Autodesk Inventor part; units mm, degrees
(part 2 of 2)
sketch "Sketch52" plane through (68.046336, 24.150723, -1) normal (0, 0.487547, 0.8730967) x (1, 0, 0)
  line L0 (-26.764269, 47.731417) -> (110.67345, 47.731417)
  line L1 (11.777064, 45.962688) -> (24.325703, 45.962688)
  line L2 (24.325703, 9.021095) -> (11.777064, 9.021095)
  line L3 (11.777064, 45.962688) -> (24.325703, 45.962688)
  line L4 (24.325703, 9.021095) -> (11.777064, 9.021095)
  line L5 (14.714671, 39.847676) -> (21.539975, 39.847676)
  line L6 (21.539975, 15.345043) -> (14.712852, 15.345043)
  line L7 (6.346286, 40.416065) -> (11.777064, 45.962688)
  line L8 (24.325703, 45.962688) -> (29.996181, 40.410641)
  line L9 (6.346286, 14.669312) -> (11.777064, 9.021095)
  line L10 (24.325703, 9.021095) -> (29.850784, 14.664032)
  line L11 (12.768778, 17.248514) -> (14.712852, 15.345043)
  line L12 (21.539975, 15.345043) -> (23.571588, 17.250974)
  line L13 (12.768778, 37.860275) -> (14.714671, 39.847676)
  line L14 (21.539975, 39.847676) -> (23.571588, 37.858494)
  line L15 (24.325703, 45.962688) -> (11.777064, 45.962688)
  line L16 (24.675506, 46.319952) -> (30.497659, 40.619399)
  line L17 (5.846286, 40.620088) -> (11.566859, 46.462688)
  line L18 (11.566859, 46.462688) -> (24.529447, 46.462688)
  line L19 (24.529447, 46.462688) -> (24.683636, 46.311992)
  line L20 (15.169294, 5.493045) -> (27.447668, 5.493045)
  line L21 (17.779421, 36.133533) -> (23.071588, 36.133533)
  line L22 (24.529447, 46.462688) -> (33.660701, 37.522418)
  line L23 (5.846286, 14.46793) -> (14.475665, 5.493045)
  line L24 (14.475665, 5.493045) -> (15.169294, 5.493045)
  line L25 (27.447668, 5.493045) -> (33.668767, 11.00658)
  line L26 (40.880024, 36.633533) -> (40.880024, 36.606569)
  line L27 (17.779421, 36.133533) -> (16.268028, 34.718457)
  line L28 (3.760683, 48.300062) -> (70.974232, 48.300062) construction
  line L29 (70.974232, 48.300062) -> (70.974232, 2.785373) construction
  line L30 (70.974232, 2.785373) -> (3.760683, 2.785373) construction
  line L31 (3.760683, 2.785373) -> (3.760683, 48.300062) construction
  line L32 (5.846286, 29.443989) -> (7.926263, 27.407454)
  line L33 (7.926263, 27.407454) -> (5.846286, 25.283108)
  line L34 (27.432742, 27.4203) -> (29.937267, 29.97825)
  line L35 (27.432742, 27.4203) -> (29.909129, 24.995634)
  line L36 (6.346286, 29.654194) -> (8.633331, 27.414916)
  line L37 (5.846286, 40.620088) -> (5.846286, 29.443989)
  line L38 (5.846286, 25.283108) -> (5.846286, 14.46793)
  line L39 (6.346286, 29.654194) -> (6.346286, 40.416065)
  line L40 (6.346286, 14.669312) -> (6.346286, 25.079086)
  line L41 (8.633331, 27.414916) -> (6.346286, 25.079086)
  line L42 (14.714671, 39.847676) -> (21.539975, 39.847676)
  line L43 (21.539975, 15.345043) -> (14.714671, 15.345043)
  line L44 (14.714671, 30.323192) -> (21.539975, 30.323192)
  line L45 (21.539975, 24.068485) -> (14.714671, 24.068485)
  line L46 (14.714671, 30.323192) -> (12.768778, 32.228443)
  line L47 (21.539975, 30.323192) -> (23.571588, 32.398142)
  line L48 (14.714671, 24.068485) -> (12.768778, 22.081084)
  line L49 (21.539975, 24.068485) -> (23.571588, 21.955529)
  line L50 (23.071588, 32.602164) -> (23.071588, 36.133533)
  line L51 (16.268028, 30.823192) -> (21.32977, 30.823192)
  line L52 (21.32977, 30.823192) -> (23.071588, 32.602164)
  line L53 (12.768778, 22.077314) -> (12.768778, 22.081084)
  line L54 (12.768778, 32.228443) -> (12.768778, 32.753075)
  line L55 (12.768778, 17.248514) -> (12.768778, 22.081084)
  line L56 (12.768778, 32.228443) -> (12.768778, 37.860275)
  line L57 (23.571588, 37.858494) -> (23.571588, 32.398142)
  line L58 (23.571588, 21.955529) -> (23.571588, 17.250974)
  line L59 (16.268028, 30.823192) -> (16.268028, 34.718457)
  line L60 (17.779421, 21.258019) -> (23.071588, 21.258019)
  line L61 (17.779421, 21.258019) -> (16.268028, 19.842942)
  line L62 (16.268028, 15.947677) -> (21.32977, 15.947677)
  line L63 (21.32977, 15.947677) -> (23.071588, 17.72665)
  line L64 (16.268028, 15.947677) -> (16.268028, 19.842942)
  line L65 (16.268028, 15.947677) -> (16.268028, 19.842942)
  line L66 (23.071588, 21.258019) -> (23.071588, 17.72665)
  line L67 (31.159581, 23.771299) -> (33.66563, 21.31759)
  line L68 (33.664106, 26.329248) -> (31.159581, 23.771299)
  line L69 (33.668767, 11.00658) -> (33.66563, 21.31759)
  line L70 (33.664106, 26.329248) -> (33.660701, 37.522418)
  line L71 (29.996181, 40.410641) -> (29.937267, 29.97825)
  line L72 (29.909129, 24.995634) -> (29.850784, 14.664032)
  line L73 (43.97433, 21.987313) -> (43.974311, 21.991083)
  line L74 (37.449269, 37.37978) -> (37.449269, 40.416067)
  line L75 (43.909742, 37.37978) -> (37.449269, 37.37978)
  line L76 (36.953115, 37.379779) -> (40.161952, 34.23796)
  line L77 (40.161952, 34.23796) -> (47.408991, 34.23796)
  line L78 (47.408991, 34.753319) -> (47.408991, 34.23796)
  line L79 (47.408991, 34.753319) -> (48.88625, 36.133533)
  line L80 (48.88625, 36.133533) -> (54.178417, 36.133533)
  line L81 (54.178417, 36.133533) -> (54.178417, 32.602164)
  line L82 (54.678417, 37.858494) -> (54.678417, 32.398142)
  line L83 (52.646804, 39.847676) -> (54.678417, 37.858494)
  line L84 (45.8215, 39.847676) -> (52.646804, 39.847676)
  line L85 (43.909742, 37.895138) -> (45.8215, 39.847676)
  line L86 (43.909742, 37.895138) -> (43.909742, 37.37978)
  line L87 (36.953115, 40.620088) -> (36.953115, 37.379779)
  line L88 (36.953115, 40.620088) -> (42.673691, 46.462691)
  line L89 (42.880047, 45.962689) -> (37.449269, 40.416067)
  line L90 (42.673691, 46.462691) -> (55.636273, 46.462691)
  ellipse E0 centre (41.918663, 54.676342) end of major axis (43.418663, 54.676342) minor radius 0.731321
  line L91 (42.880047, 45.962689) -> (55.428686, 45.962689)
  line L92 (26.413444, 60.77068) -> (58.413444, 60.77068)
  line L93 (55.428686, 45.962689) -> (61.099164, 40.410643)
  line L94 (55.636273, 46.462691) -> (64.767394, 37.522279)
  line L95 (61.099164, 40.410643) -> (61.099164, 29.978085)
  line L96 (64.767394, 37.522279) -> (64.767394, 26.329108)
  line L97 (61.099164, 29.978085) -> (55.300317, 23.988246)
  line L98 (64.767394, 26.329108) -> (59.830797, 21.22992)
  line L99 (55.300317, 23.988246) -> (45.910182, 23.988246)
  line L100 (59.830797, 21.22992) -> (48.911426, 21.22992)
  line L101 (45.910182, 23.988246) -> (43.97433, 21.987313)
  line L102 (48.911426, 21.22992) -> (47.471798, 19.741893)
  line L103 (43.97433, 21.987313) -> (43.97433, 17.158512)
  line L104 (47.471798, 19.741893) -> (47.471798, 15.850429)
  line L105 (43.97433, 17.158512) -> (45.918411, 15.25505)
  line L106 (47.471798, 15.850429) -> (61.143322, 15.850429)
  line L107 (61.060189, 15.25505) -> (45.918411, 15.25505)
  line L108 (61.060189, 15.25505) -> (61.060189, 9.021005)
  line L109 (61.143322, 15.850429) -> (64.868674, 12.202883)
  line L110 (64.868674, 12.202883) -> (64.868674, 5.510434)
  line L111 (61.060189, 9.021005) -> (37.453115, 9.021005)
  line L112 (64.868674, 5.510434) -> (40.538917, 5.510434)
  line L113 (69.848141, 4.102168) -> (69.848141, -14.686273)
  line L114 (36.935591, 9.038395) -> (40.538917, 5.510434)
  line L115 (36.935591, 25.300498) -> (36.935591, 9.038395)
  line L116 (37.453115, 25.079086) -> (37.453115, 9.021005)
  line L117 (36.935591, 25.300498) -> (42.433502, 30.823192)
  line L118 (42.673688, 30.323192) -> (37.453115, 25.079086)
  line L119 (42.433502, 30.823192) -> (52.436599, 30.823192)
  line L120 (52.646804, 30.323192) -> (42.673688, 30.323192)
  line L121 (52.436599, 30.823192) -> (54.178417, 32.602164)
  line L122 (54.678417, 32.398142) -> (52.646804, 30.323192)
  point P0 (-68.046336, -21.573465)
  point P1 (24.675164, 46.320287)
  point P2 (65.459194, 32.753075)
  point P3 (65.459194, 32.753075)
  point P4 (30.502764, 40.625302)
  point P5 (12.768778, 22.077314)
  dimension "d185" = 0.5
  dimension "d227" = 0.5
  dimension "d228" = 0.5
  constraints: 232 end point, 34 parallel, 16 horizontal, 9 vertical, 6 perpendicular, 4 point on line, 1 coincident, 5 other
  measures "d185" distance between parallel lines of L8 L16
  measures "d227" distance between parallel lines of L44 L51
  measures "d228" distance between parallel lines of L47 L52
extrude "Extrusion52" cut sketch "Sketch52" against normal blind 0.5 contours L5 L14 L57 L47 L44 L46 L54 L56 L13 | L6 L11 L55 L53 L48 L45 L49 L58 L12 | L16 L22 L70 L68 L67 L69 L25 L20 L24 L23 L38 L33 L32 L37 L17 L18 L19 | L87 L88 L90 L94 L96 L98 L100 L102 L104 L106 L109 L110 L112 L114 L115 L117 L119 L121 L81 L80 L79 L78 L77 L76
body "Solid1"
